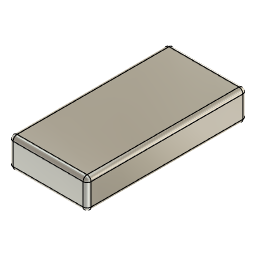
Battery (Autodesk Fusion 360 design; units mm, degrees)
Autodesk Fusion 360 part; units mm, degrees
sketch "草图1" plane through (0, 0, 0) normal (0, 0, 1) x (1, 0, 0)
  line L0 (9.75, 20) -> (-9.75, 20)
  line L1 (-9.75, 20) -> (-9.75, -20)
  line L2 (-9.75, -20) -> (9.75, -20)
  line L3 (9.75, -20) -> (9.75, 20)
  line L4 (9.75, 20) -> (-9.75, -20) construction
  line L5 (-9.75, 20) -> (9.75, -20) construction
  dimension "d1" = 19.5
  dimension "d2" = 40
  constraint horizontal L0
  constraint perpendicular L0 L1
  constraint parallel L0 L2
  constraint parallel L1 L3
  constraint coincident L4 origin
  constraint coincident L5 origin
  measures "d1" distance of L1 L3
  measures "d2" distance of L0 L2
extrude "拉伸1" add sketch "草图1" along normal mid plane 7.5
fillet "圆角1" radius 1 1 edges at (-9.75, 0, 3.75) 5 faces at (3.25, -6.6667, 3.75) (-9.75, -6.6667, 1.25) (-3.25, -20, -1.25) (9.75, -6.6667, -1.25) (-3.25, 20, 1.25)
